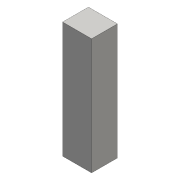
# Autodesk Inventor part: Base
Saved by Autodesk Inventor 2016 (Build 200138000, 138)
## iProperties
Created: 2020-10-21
Part Number: Base
Material: Generic
Document SubType Name: Modeling
Designer: extract
Density: 1 g/cm^3
Appearance: Default
Author: extract
Autodesk Inventor part; units mm, degrees
ref_plane "YZ Plane" through (0, 0, 0) normal (1, 0, 0) x (0, 1, 0)
ref_plane "XZ Plane" through (0, 0, 0) normal (0, 1, 0) x (-1, 0, 0)
ref_plane "XY Plane" through (0, 0, 0) normal (0, 0, 1) x (1, 0, 0)
sketch "Sketch1" plane through (0, 0, 0) normal (0, 1, 0) x (-1, 0, 0)
  line L0 (-125, 500) -> (125, 500)
  line L1 (125, 500) -> (125, -500)
  line L2 (125, -500) -> (-125, -500)
  line L3 (-125, -500) -> (-125, 500)
  line L4 (-125, 500) -> (125, -500) construction
  line L5 (125, 500) -> (-125, -500) construction
  point P0 (0, 0)
  dimension "d0" = 250
  dimension "d1" = 1000
  constraints: 12 end point, 2 midpoint, 2 parallel, 1 horizontal, 1 perpendicular
  measures "d0" distance of L1.end L2.end
  measures "d1" distance of L0.end L1.end
extrude "Extrusion1" add sketch "Sketch1" along normal blind 222.5
body "Solid1"
